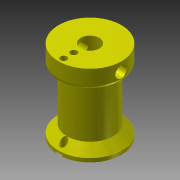
# Autodesk Inventor part: PULLEY
Saved by Autodesk Inventor 2013 (Build 170138000, 138)
## iProperties
Created: 2013-11-27
Part Number: PULLEY
Material: Generic
Document SubType Name: Modeling
Designer: employee
Density: 1 g/cm^3
Author: employee
Autodesk Inventor part; units mm, degrees
ref_plane "YZ Plane" through (0, 0, 0) normal (1, 0, 0) x (0, 1, 0)
ref_plane "XZ Plane" through (0, 0, 0) normal (0, 1, 0) x (-1, 0, 0)
ref_plane "XY Plane" through (0, 0, 0) normal (0, 0, 1) x (1, 0, 0)
sketch "Sketch1" plane through (0, 0, 0) normal (0, 0, 1) x (1, 0, 0)
  circle A0 centre (0, 0) radius 6.25
  circle A1 centre (0, 0) radius 2.525
  dimension "d0" = 12.5
  dimension "d2" = 5.05
  constraints: 2 centre point, 2 coincident
  measures "d0" diameter of A0
  measures "d2" diameter of A1
extrude "Extrusion1" add sketch "Sketch1" along normal blind 22
sketch "Sketch3" plane through (0, 0, 22) normal (0, 0, 1) x (1, 0, 0)
  circle A0 centre (0, 0) radius 2.525 projected
  circle A1 centre (0, 0) radius 6.25 projected
  circle A2 centre (0, 0) radius 8.525
  dimension "d9" = 6
  constraints: 1 centre point, 1 coincident
  measures "d9" radial gap between concentric circles of A2 A0
extrude "Extrusion3" add sketch "Sketch3" against normal blind 5 contours A2
sketch "Sketch4" plane through (0, 0, 0) normal (1, 0, 0) x (0, 1, 0)
  line L0 (-2.525, 22) -> (-2.525, 0) projected
  line L1 (-2.525, 0) -> (-6.25, 0) projected
  line L2 (-6.25, 0) -> (-6.25, 17) projected
  line L3 (-6.25, 17) -> (-8.525, 17) projected
  line L4 (-8.525, 17) -> (-8.525, 22) projected
  line L5 (-8.525, 22) -> (-2.525, 22) projected
  line L6 (2.525, 0) -> (2.525, 22) projected
  line L7 (2.525, 22) -> (8.525, 22) projected
  line L8 (8.525, 22) -> (8.525, 17) projected
  line L9 (8.525, 17) -> (6.25, 17) projected
  line L10 (6.25, 17) -> (6.25, 0) projected
  line L11 (6.25, 0) -> (2.525, 0) projected
  circle A0 centre (0, 19.5) radius 1.525
  point P0 (0, 0)
  point P1 (8.525, 19.5)
  dimension "d13" = 3.05
  constraints: 1 centre point, 1 horizontal alignment, 1 midpoint, 1 vertical alignment
  measures "d13" diameter of A0
extrude "Extrusion4" cut sketch "Sketch4" along normal through all both and the other way through all contours A0
sketch "Sketch6" plane through (0, 0, 0) normal (0, 0, -1) x (-1, 0, 0)
  circle A0 centre (0, 0) radius 6.25 projected
  circle A1 centre (0, 0) radius 8.525 projected
extrude "Extrusion6" add sketch "Sketch6" against normal blind 1
chamfer "Chamfer1" distance 2.25 angle 45 1 edges at (-6.25, 0, 1)
sketch "Sketch5" plane through (0, 0, 22) normal (0, 0, 1) x (1, 0, 0)
  circle A0 centre (0, 0) radius 8.525 projected
  circle A1 centre (0, 0) radius 2.525 projected
  circle A2 centre (0, 0) radius 6.25 projected
  circle A3 centre (0, -7.125) radius 0.875
  circle A4 centre (0, -4.3875) radius 0.875
  line L0 (0, -6.25) -> (0, -2.525)
  dimension "d20" = 1.75
  dimension "d17" = 1.75
  constraints: 4 vertical alignment, 2 end point, 1 centre point, 1 midpoint, 1 vertical, 4 other
  measures "d17" diameter of A4
extrude "Extrusion5" cut sketch "Sketch5" against normal through all contours A3 | A4 L0 | L0 A4
fillet "Fillet1" radius 1 1 edges at (-8.525, 0, 17)
sketch "Sketch7" plane through (0, 0, 0) normal (0, 0, -1) x (-1, 0, 0)
  circle A0 centre (0, -7.125) radius 0.875 projected
  circle A1 centre (0, -4.3875) radius 0.875 projected
  circle A2 centre (0, 0) radius 8.525 projected
  line L0 (-0.875, 8.525) -> (0.875, 8.525)
  line L1 (0.875, 8.525) -> (0.875, -8.525)
  line L2 (0.875, -8.525) -> (-0.875, -8.525)
  line L3 (-0.875, -8.525) -> (-0.875, 8.525)
  constraints: 8 end point, 4 tangent, 2 parallel, 1 horizontal, 1 perpendicular
extrude "Extrusion7" cut sketch "Sketch7" against normal blind 0.5 contours L1 A2 L3 A0 | A0 L3 A1 L1 | A1 L3 A2 L1 | L1 L2 A2 | A2 L2 L3 | A2 L0 L1 | L3 L0 A2
body "Solid1"
